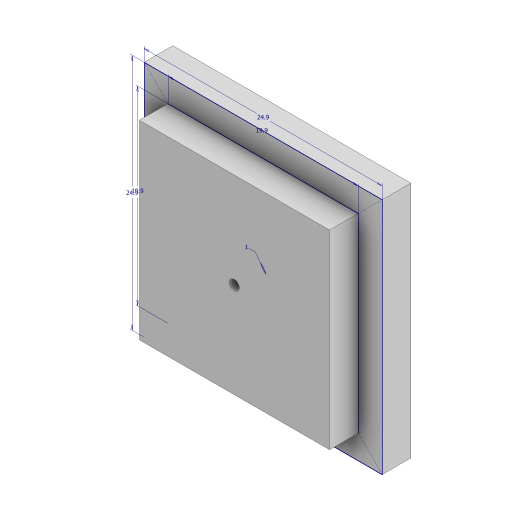
# Autodesk Inventor part: Large-cuvette-cap-25mm
Saved by Autodesk Inventor 2023 (Build 270158000, 158)
## iProperties
Created: 2023-04-14
Part Number: Large-cuvette-cap-25mm
Material: Generic
Document SubType Name: Modeling
Designer: nvladi
Density: 1 g/cm^3
Appearance: Default
Author: nvladi
Autodesk Inventor part; units mm, degrees
ref_plane "YZ Plane" through (0, 0, 0) normal (1, 0, 0) x (0, 1, 0)
ref_plane "XZ Plane" through (0, 0, 0) normal (0, 1, 0) x (-1, 0, 0)
ref_plane "XY Plane" through (0, 0, 0) normal (0, 0, 1) x (1, 0, 0)
sketch "Sketch1" plane through (0, 0, 0) normal (0, 0, 1) x (1, 0, 0)
  line L0 (9.95, -9.95) -> (-9.95, -9.95)
  line L1 (-9.95, -9.95) -> (-9.95, 9.95)
  line L2 (-9.95, 9.95) -> (9.95, 9.95)
  line L3 (9.95, 9.95) -> (9.95, -9.95)
  line L4 (9.95, -9.95) -> (-9.95, 9.95) construction
  line L5 (-9.95, -9.95) -> (9.95, 9.95) construction
  circle A0 centre (0, 0) radius 0.5
  line L6 (12.45, -12.45) -> (-12.45, -12.45)
  line L7 (-12.45, -12.45) -> (-12.45, 12.45)
  line L8 (-12.45, 12.45) -> (12.45, 12.45)
  line L9 (12.45, 12.45) -> (12.45, -12.45)
  line L10 (12.45, -12.45) -> (-12.45, 12.45) construction
  line L11 (-12.45, -12.45) -> (12.45, 12.45) construction
  dimension "d2" = 19.9
  dimension "d3" = 19.9
  dimension "d4" = 1
  dimension "d5" = 24.9
  dimension "d6" = 24.9
  constraints: 24 end point, 4 midpoint, 4 parallel, 2 horizontal, 2 perpendicular, 1 centre point, 1 coincident
  measures "d2" distance between parallel lines of L3 L1
  measures "d3" distance between parallel lines of L0 L2
  measures "d4" diameter of A0
  measures "d5" distance of L7.end L8.end
  measures "d6" distance of L6.end L7.end
extrude "Extrusion1" add sketch "Sketch1" along normal blind 3 contours L0 L1 L2 L3
extrude "Extrusion2" add sketch "Sketch1" against normal blind 3 contours L0 L1 L2 L3 | L6 L7 L8 L9
body "Solid1"
